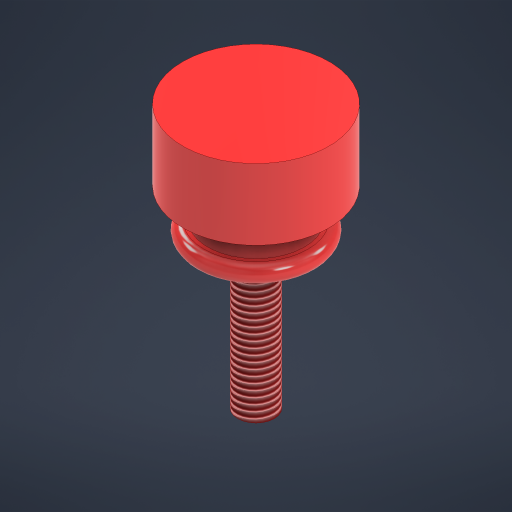
# Autodesk Inventor part: M3_Safety_Knob
Saved by Autodesk Inventor 2024.1 (Build 281209000, 209)
## iProperties
Created: 2023-12-07
Part Number: M3_Safety_Knob
Material: Aluminum 6061
Document SubType Name: Modeling
Designer: dzw04
Density: 2.7 g/cm^3
Appearance: Light Red
Author: dzw04
Autodesk Inventor part; units mm, degrees
ref_plane "YZ Plane" through (0, 0, 0) normal (1, 0, 0) x (0, 1, 0)
ref_plane "XZ Plane" through (0, 0, 0) normal (0, 1, 0) x (-1, 0, 0)
ref_plane "XY Plane" through (0, 0, 0) normal (0, 0, 1) x (1, 0, 0)
sketch "Sketch1" plane through (0, 0, 0) normal (0, 1, 0) x (-1, 0, 0)
  circle A0 centre (0, 0) radius 6
  dimension "d0" = 12
  constraints: 1 centre point, 1 coincident
  measures "d0" diameter of A0
extrude "Extrusion1" add sketch "Sketch1" along normal blind 5.8
sketch "Sketch2" plane through (0, 0, 0) normal (0, -1, 0) x (1, 0, 0)
  circle A0 centre (0, 0) radius 3.95
  dimension "d3" = 7.9
  constraints: 1 centre point, 1 coincident
  measures "d3" diameter of A0
extrude "Extrusion2" add sketch "Sketch2" along normal blind 2.4
sketch "Sketch3" plane through (0, -2.4, 0) normal (0, -1, 0) x (1, 0, 0)
  circle A0 centre (0, 0) radius 4.95
  dimension "d6" = 9.9
  constraints: 1 centre point, 1 coincident
  measures "d6" diameter of A0
extrude "Extrusion3" add sketch "Sketch3" along normal blind 1.4
fillet "Fillet1" radius 0.7 2 edges at (-4.95, -2.4, 0) (-4.95, -3.8, 0)
sketch "Sketch4" plane through (0, -3.8, 0) normal (0, -1, 0) x (1, 0, 0)
  circle A0 centre (0, 0) radius 1.5
  dimension "d10" = 3
  constraints: 1 centre point, 1 coincident
  measures "d10" diameter of A0
extrude "Extrusion4" add sketch "Sketch4" along normal blind 12
thread "Thread1" size "M3x0.5" class "6g" standard "ANSI Metric M Profile" full length
body "Solid1"
